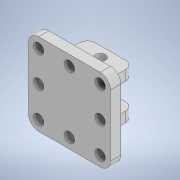
# Autodesk Inventor part: hinge
Saved by Autodesk Inventor 2021 (Build 250183000, 183)
## iProperties
Created: 2021-04-17
Part Number: hinge
Material: Generic
Document SubType Name: Modeling
Designer: gfellows
Density: 1 g/cm^3
Appearance: Default
Author: gfellows
Autodesk Inventor part; units mm, degrees
ref_plane "YZ Plane" through (0, 0, 0) normal (1, 0, 0) x (0, 1, 0)
ref_plane "XZ Plane" through (0, 0, 0) normal (0, 1, 0) x (-1, 0, 0)
ref_plane "XY Plane" through (0, 0, 0) normal (0, 0, 1) x (1, 0, 0)
ref_plane "Work Plane1" through (-192, 24, -212) normal (0, 0, -1) x (-1, 0, 0)
sketch "Sketch1" plane through (-192, 24, -212) normal (0, 0, -1) x (-1, 0, 0)
  circle A0 centre (-32, -8) radius 2 projected
  arc A1 (-30.5858, -33.4142) -> (-33.4142, -30.5858) centre (-32, -32) ccw projected
  arc A2 (-6.5858, -33.4142) -> (-9.4142, -30.5858) centre (-8, -32) ccw projected
  circle A3 centre (-8, -8) radius 2 projected
  circle A4 centre (-32, -32) radius 2
  circle A5 centre (-8, -32) radius 2
  circle A6 centre (-8, -8) radius 2
  circle A7 centre (-32, -8) radius 2
  circle A8 centre (-32, -8) radius 4
  circle A9 centre (-8, -8) radius 4
  circle A10 centre (-8, -32) radius 4
  circle A11 centre (-32, -32) radius 4
  line L0 (-36, -8) -> (-36, -32)
  line L1 (-32, -36) -> (-8, -36)
  line L2 (-4, -32) -> (-4, -8)
  line L3 (-8, -4) -> (-32, -4)
  circle A12 centre (-32, -20) radius 2
  line L4 (-32, -8) -> (-32, -20) construction
  line L5 (-32, -20) -> (-32, -32) construction
  circle A13 centre (-8, -20) radius 2
  circle A14 centre (-20, -8) radius 2
  line L6 (-32, -8) -> (-20, -8) construction
  line L7 (-20, -8) -> (-8, -8) construction
  circle A15 centre (-20, -32) radius 2
  point P0 (-9.4142, -30.5858)
  point P1 (-33.4142, -30.5858)
  dimension "d0" = 2
  dimension "d1" = 2
  dimension "d2" = 2
  dimension "d3" = 2
  dimension "d31" = 4
  dimension "d32" = 4
  dimension "d33" = 4
  dimension "d34" = 4
  dimension "d35" = 4
  constraints: 16 end point, 10 centre point, 8 point on circle, 8 tangent, 4 coincident, 3 horizontal alignment, 3 vertical alignment, 2 collinear, 2 concentric, 2 horizontal, 2 vertical, 6 other
  measures "d0" radial gap between concentric circles of A0 A8
  measures "d1" radial gap between concentric circles of A3 A9
  measures "d31" diameter of A12
  measures "d32" diameter of A13
  measures "d33" diameter of A6
  measures "d34" diameter of A14
  measures "d35" diameter of A15
extrude "Extrusion1" add sketch "Sketch1" along normal blind 4
sketch "Sketch2" plane through (-192, 24, -216) normal (0, 0, -1) x (-1, 0, 0)
  line L0 (-36, -8) -> (-36, -32) projected
  line L1 (-4, -32) -> (-4, -8) projected
  line L2 (-4, -32) -> (-4, -8) projected
  line L3 (-36, -11) -> (-4, -11)
  line L4 (-4, -11) -> (-4, -29)
  line L5 (-4, -29) -> (-36, -29)
  line L6 (-36, -29) -> (-36, -11)
  circle A0 centre (-32, -8) radius 2 projected
  circle A1 centre (-8, -8) radius 2 projected
  circle A2 centre (-8, -32) radius 2 projected
  circle A3 centre (-32, -32) radius 2 projected
  line L7 (-29, -11) -> (-29, -29)
  line L8 (-11, -11) -> (-11, -29)
  point P0 (-192, -24)
  dimension "d6" = 3
  dimension "d7" = 3
  dimension "d8" = 3
  dimension "d9" = 3
  constraints: 12 end point, 6 point on line, 3 perpendicular, 2 parallel, 1 horizontal
  measures "d6" distance from line of L5 A3.centre
  measures "d7" distance from line of A0.centre L3
  measures "d8" distance from line of L8 A1.centre
  measures "d9" distance from line of L7 A0.centre
extrude "Extrusion2" add sketch "Sketch2" along normal blind 12 contours L3 L8 L5 L7
sketch "Sketch3" plane through (-181, -5, -216) normal (-1, 0, 0) x (0, 0, 1)
  line L0 (0, 18) -> (0, 0) projected
  line L1 (0, 18) -> (-12, 18) projected
  line L2 (-12, 0) -> (-12, 18) projected
  line L3 (0, 0) -> (-12, 0) projected
  line L4 (-12, 18) -> (-12, 0) projected
  line L5 (0, 21) -> (0, -3) projected
  line L6 (-12, 14) -> (0, 14)
  line L7 (0, 14) -> (0, 4)
  line L8 (0, 4) -> (-12, 4)
  line L9 (-12, 4) -> (-12, 14)
  point P0 (216, 5)
  point P1 (-12, 4)
  point P2 (0, 4)
  point P3 (0, 14)
  dimension "d12" = 4
  dimension "d13" = 4
  constraints: 8 end point, 2 parallel, 2 point on line, 1 horizontal, 1 perpendicular
  measures "d12" distance between parallel lines of L1 L6
  measures "d13" distance between parallel lines of L3 L8
extrude "Extrusion3" cut sketch "Sketch3" against normal through all contours L0 L8 L2 L6
fillet "Fillet1" radius 3.175 8 edges at (-181, 11, -228) (-163, 11, -228) (-181, 11, -216) (-163, 11, -216) (-163, -3, -216) (-163, -3, -228) (-181, -3, -228) (-181, -3, -216)
sketch "Sketch4" plane through (-184.175, 13, -216) normal (0, 1, 0) x (1, 0, 0)
  arc A0 (21.175, 8.825) -> (18, 12) centre (18, 8.825) ccw projected
  line L0 (6.35, 12) -> (18, 12) projected
  arc A1 (6.35, 12) -> (3.175, 8.825) centre (6.35, 8.825) ccw projected
  line L1 (3.175, 3.175) -> (3.175, 8.825) projected
  arc A2 (0, 0) -> (3.175, 3.175) centre (0, 3.175) ccw projected
  line L2 (24.35, 0) -> (0, 0) projected
  arc A3 (21.175, 3.175) -> (24.35, 0) centre (24.35, 3.175) ccw projected
  line L3 (21.175, 3.175) -> (21.175, 8.825) projected
  circle A4 centre (12.175, 8) radius 2
  point P0 (184.175, -216)
  dimension "d17" = 4
  dimension "d18" = 18
  dimension "d19" = 9
  dimension "d20" = 12
  dimension "d21" = 8
  constraints: 1 centre point
  measures "d17" diameter of A4
  measures "d18" distance between parallel lines of L1 L3
  measures "d19" distance from line of L1 A4.centre
  measures "d20" distance between parallel lines of L2 L0
  measures "d21" distance from line of L2 A4.centre
extrude "Extrusion4" cut sketch "Sketch4" against normal through all contours A4
sketch "Sketch5" plane through (-192, 24, -216) normal (0, 0, -1) x (-1, 0, 0)
  line L0 (-7.825, -29) -> (-32.175, -29) projected
  line L1 (-32.175, -25) -> (-32.175, -29) projected
  line L2 (-7.825, -25) -> (-32.175, -25) projected
  line L3 (-7.825, -29) -> (-7.825, -25) projected
  line L4 (-32.175, -11) -> (-7.825, -11) projected
  line L5 (-7.825, -15) -> (-7.825, -11) projected
  line L6 (-7.825, -15) -> (-32.175, -15) projected
  line L7 (-32.175, -11) -> (-32.175, -15) projected
  line L8 (-36, -8) -> (-36, -32) projected
  arc A0 (-36, -32) -> (-32, -36) centre (-32, -32) ccw projected
  line L9 (-32, -36) -> (-8, -36) projected
  arc A1 (-8, -36) -> (-4, -32) centre (-8, -32) ccw projected
  line L10 (-4, -32) -> (-4, -8) projected
  arc A2 (-4, -8) -> (-8, -4) centre (-8, -8) ccw projected
  line L11 (-8, -4) -> (-32, -4) projected
  arc A3 (-32, -4) -> (-36, -8) centre (-32, -8) ccw projected
  circle A4 centre (-8, -32) radius 2 projected
  circle A5 centre (-32, -32) radius 2 projected
  circle A6 centre (-32, -8) radius 2 projected
  circle A7 centre (-8, -8) radius 2 projected
  circle A8 centre (-32, -8) radius 4
  circle A9 centre (-8, -8) radius 4
  circle A10 centre (-8, -32) radius 2 projected
  circle A11 centre (-8, -32) radius 4
  circle A12 centre (-32, -32) radius 4
  point P0 (-192, -24)
  dimension "d24" = 8
  dimension "d25" = 8
  dimension "d26" = 8
  dimension "d27" = 8
  constraints: 4 centre point, 4 coincident
  measures "d24" diameter of A8
  measures "d25" diameter of A9
  measures "d26" diameter of A11
  measures "d27" diameter of A12
extrude "Extrusion5" cut sketch "Sketch5" along normal blind 25.4 contours L3 A11 A1 L0 | L0 A11 L3 | A12 A0 L1 L0 | L0 L1 A12 | A9 L5 L4 A2 | A9 L4 L5 | A3 A8 L4 L7 | L7 L4 A8 | A4 | A5 | A6 | A7
sketch "Sketch6" plane through (-177.825, 13, -228) normal (0, 1, 0) x (1, 0, 0)
  circle A0 centre (5.825, -4) radius 2 projected
  circle A1 centre (5.825, -4) radius 4
  point P0 (177.825, -228)
  dimension "d30" = 8
  constraints: 1 centre point, 1 coincident
  measures "d30" diameter of A1
equation "\"d0\" = d1"
equation "\"d2\" = d1"
equation "\"d3\" = d1"
equation "\"d19\" = 0.5 * d18"
equation "\"d21\" = 0.666667 * d20"
equation "\"d25\" = d24"
equation "\"d26\" = d25"
equation "\"d27\" = d24"
body "Solid1"
